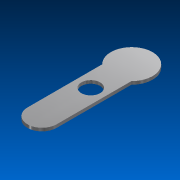
# Autodesk Inventor part: Terminal 1
Saved by Autodesk Inventor 2013 (Build 170138000, 138)
## iProperties
Created: 2012-05-07
Project: 2.1mm DC Power Socket
Material: Brass, Soft Yellow
Description: Terminal 1
Document SubType Name: Modeling
Designer: sdarley
Density: 1 g/cm^3
Title: Terminal 1
Author: sdarley
Revision Number: 1
Autodesk Inventor part; units mm, degrees
ref_plane "YZ Plane" through (0, 0, 0) normal (1, 0, 0) x (0, 1, 0)
ref_plane "XZ Plane" through (0, 0, 0) normal (0, 1, 0) x (-1, 0, 0)
ref_plane "XY Plane" through (0, 0, 0) normal (0, 0, 1) x (1, 0, 0)
sketch "Sketch1" plane through (0, 0, 0) normal (0, 0, 1) x (1, 0, 0)
  arc A0 (1.4, -1.4283) -> (-1.4, -1.4283) centre (0, 0) ccw
  line L0 (-1.4, -1.4283) -> (-1.4, -10)
  line L1 (-1.4, -10) -> (1.4, -10)
  line L2 (1.4, -10) -> (1.4, -1.4283)
  point P0 (0, -10)
  dimension "d0" = 4
  dimension "d1" = 2.8
  dimension "d2" = 12
  constraints: 6 end point, 2 point on circle, 1 centre point, 1 coincident, 1 midpoint, 1 parallel, 1 perpendicular, 1 vertical, 1 vertical alignment
  measures "d0" diameter of A0
  measures "d1" distance of L0.end L1.end
extrude "Extrusion1" add sketch "Sketch1" along normal blind 0.3
fillet "Fillet1" radius 1.4 2 edges at (1.4, -10, 0.15) (-1.4, -10, 0.15)
sketch "Sketch2" plane through (0, 0, 0.3) normal (0, 0, 1) x (1, 0, 0)
  circle A0 centre (0, -3.9283) radius 0.9
  point P0 (1.4, -1.4283)
  dimension "d6" = 1.8
  dimension "d7" = 2.5
  constraints: 1 centre point
  measures "d6" diameter of A0
  measures "d7" vertical distance of A0.centre point (1.4, -1.428)
extrude "Extrusion2" cut sketch "Sketch2" against normal through all
body "Solid1"
